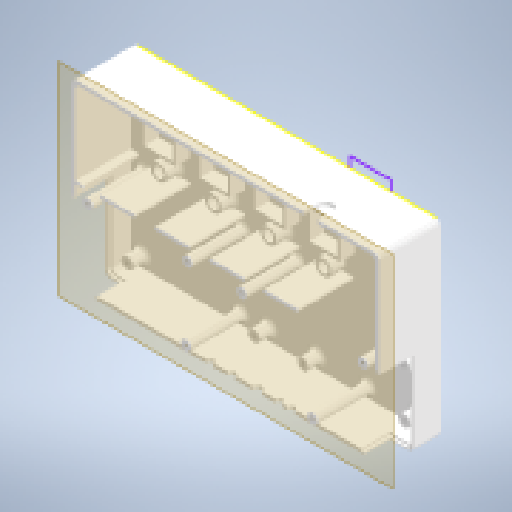
# Autodesk Inventor part: RV_ES_Bottom
Saved by Autodesk Inventor 2024.2 (Build 282272000, 272)
## iProperties
Created: 2023-07-31
Part Number: RV_ES_Bottom
Material: PC/ABS Plastic
Document SubType Name: Modeling
Designer: atrus
Density: 0.357273 g/cm^3
Appearance: Smooth - White
Mass: 71.7319 g
Surface Area: 1331.28 cm^2
Volume: 200.776 cm^3
Author: atrus
Autodesk Inventor part; units mm, degrees
ref_plane "YZ Plane" through (0, 0, 0) normal (1, 0, 0) x (0, 1, 0)
sketch "Sketch1" plane through (0, 0, 0) normal (0, 0, 1) x (1, 0, 0)
  line L0 (0, 0) -> (215.9, 0)
  line L1 (215.9, 0) -> (215.9, 132.08)
  line L2 (215.9, 132.08) -> (0, 132.08)
  line L3 (0, 132.08) -> (0, 0)
  dimension "d0" = 215.9
  dimension "d1" = 132.08
  constraints: 8 end point, 2 parallel, 1 horizontal, 1 perpendicular
  measures "d0" distance of L1.end L2.end
  measures "d1" distance of L0.end L1.end
extrude "BasePlate" add sketch "Sketch1" along normal blind 4
sketch "Sketch2" plane through (0, 0, 4) normal (0, 0, 1) x (1, 0, 0)
  circle A0 centre (10.16, 10.16) radius 1.7 construction
  circle A1 centre (99.06, 10.16) radius 1.7 construction
  circle A2 centre (133.35, 10.16) radius 1.7 construction
  circle A3 centre (204.47, 11.43) radius 1.7 construction
  circle A4 centre (156.21, 123.19) radius 1.7 construction
  circle A5 centre (123.19, 123.19) radius 1.7 construction
  circle A6 centre (80.01, 123.19) radius 1.7 construction
  circle A7 centre (46.99, 123.134) radius 1.7 construction
  circle A8 centre (10.16, 10.16) radius 4
  circle A9 centre (99.06, 10.16) radius 4
  circle A10 centre (133.35, 10.16) radius 4
  circle A11 centre (204.47, 11.43) radius 4
  circle A12 centre (156.21, 123.19) radius 4
  circle A13 centre (123.19, 123.19) radius 4
  circle A14 centre (80.01, 123.19) radius 4
  circle A15 centre (46.99, 123.134) radius 4
  circle A16 centre (8.89, 123.19) radius 1.7 construction
  circle A17 centre (8.89, 123.19) radius 4
  circle A18 centre (204.47, 44.45) radius 4
  circle A19 centre (204.47, 44.45) radius 1.7 construction
  point P0 (0, 0)
  dimension "d4" = 8
  constraints: 11 centre point, 9 equal radius, 1 coincident, 2 other
  measures "d4" diameter of A8
ref_plane "Work Plane1" through (5.1378, 6.7962, 14) normal (0, 0, 1) x (0.0000001, 1, 0)
extrude "PCB Screw Bosses" add sketch "Sketch2" along normal up to surface (10 mm away)
sketch "Sketch3" plane through (0, 0, 4) normal (0, 0, 1) x (1, 0, 0)
  line L0 (0, 0) -> (215.9, 0)
  line L1 (215.9, 0) -> (215.9, 132.08)
  line L2 (215.9, 132.08) -> (0, 132.08)
  line L3 (0, 132.08) -> (0, 0)
  line L4 (213.487, 129.667) -> (213.487, 2.413)
  line L5 (213.487, 2.413) -> (2.413, 2.413)
  line L6 (2.413, 2.413) -> (2.413, 129.667)
  line L7 (2.413, 129.667) -> (213.487, 129.667)
  point P0 (0, 132.08)
  point P1 (215.9, 0)
  dimension "d7" = 2.413
  constraints: 16 end point, 4 parallel, 2 perpendicular, 1 horizontal, 3 other
  measures "d7" distance between parallel lines of L1 L4
extrude "OuterCaseWall" add sketch "Sketch3" along normal blind 15.24
sketch "Sketch4" plane through (0, 0, 4) normal (0, 0, 1) x (1, 0, 0)
  line L0 (2.413, 129.667) -> (2.413, 2.413) projected
  line L1 (2.413, 129.667) -> (213.487, 129.667) projected
  line L2 (43.1672, 85.3312) -> (20.8152, 85.3312) construction
  line L3 (19.2531, 110.0327) -> (44.7547, 110.0327) construction
  line L4 (19.2531, 84.5311) -> (19.2531, 110.0327) construction
  line L5 (44.7547, 110.0327) -> (44.7547, 84.5311) construction
  line L6 (57.6071, 84.5311) -> (57.6071, 110.0327) construction
  line L7 (81.5212, 85.3312) -> (59.1692, 85.3312) construction
  line L8 (83.1087, 110.0327) -> (83.1087, 84.5311) construction
  line L9 (57.6071, 110.0327) -> (83.1087, 110.0327) construction
  line L10 (96.2151, 110.0327) -> (121.7167, 110.0327) construction
  line L11 (121.7167, 110.0327) -> (121.7167, 84.5311) construction
  line L12 (96.2151, 84.5311) -> (96.2151, 110.0327) construction
  line L13 (120.1292, 85.3312) -> (97.7772, 85.3312) construction
  line L14 (158.7372, 85.3312) -> (136.3852, 85.3312) construction
  line L15 (134.8231, 84.5311) -> (134.8231, 110.0327) construction
  line L16 (134.8231, 110.0327) -> (160.3247, 110.0327) construction
  line L17 (160.3247, 110.0327) -> (160.3247, 84.5311) construction
  line L18 (20.2531, 85.5311) -> (43.7547, 85.5311)
  line L19 (43.7547, 85.5311) -> (43.7547, 109.0327)
  line L20 (43.7547, 109.0327) -> (20.2531, 109.0327)
  line L21 (20.2531, 109.0327) -> (20.2531, 85.5311)
  line L22 (41.7547, 107.0327) -> (22.2531, 107.0327)
  line L23 (22.2531, 107.0327) -> (22.2531, 87.5311)
  line L24 (22.2531, 87.5311) -> (41.7547, 87.5311)
  line L25 (41.7547, 87.5311) -> (41.7547, 107.0327)
  line L26 (58.8611, 109.0327) -> (58.8611, 85.5311)
  line L27 (60.8611, 107.0327) -> (60.8611, 87.5311)
  line L28 (80.3627, 107.0327) -> (60.8611, 107.0327)
  line L29 (82.3627, 109.0327) -> (58.8611, 109.0327)
  line L30 (80.3627, 87.5311) -> (80.3627, 107.0327)
  line L31 (82.3627, 85.5311) -> (82.3627, 109.0327)
  line L32 (60.8611, 87.5311) -> (80.3627, 87.5311)
  line L33 (58.8611, 85.5311) -> (82.3627, 85.5311)
  line L34 (97.4691, 109.0327) -> (97.4691, 85.5311)
  line L35 (99.4691, 107.0327) -> (99.4691, 87.5311)
  line L36 (118.9707, 107.0327) -> (99.4691, 107.0327)
  line L37 (120.9707, 109.0327) -> (97.4691, 109.0327)
  line L38 (118.9707, 87.5311) -> (118.9707, 107.0327)
  line L39 (120.9707, 85.5311) -> (120.9707, 109.0327)
  line L40 (99.4691, 87.5311) -> (118.9707, 87.5311)
  line L41 (97.4691, 85.5311) -> (120.9707, 85.5311)
  line L42 (136.0771, 109.0327) -> (136.0771, 85.5311)
  line L43 (138.0771, 107.0327) -> (138.0771, 87.5311)
  line L44 (157.5787, 107.0327) -> (138.0771, 107.0327)
  line L45 (159.5787, 109.0327) -> (136.0771, 109.0327)
  line L46 (157.5787, 87.5311) -> (157.5787, 107.0327)
  line L47 (159.5787, 85.5311) -> (159.5787, 109.0327)
  line L48 (138.0771, 87.5311) -> (157.5787, 87.5311)
  line L49 (136.0771, 85.5311) -> (159.5787, 85.5311)
  point P0 (0, 0)
  point P1 (19.2531, 97.2819)
  dimension "d138" = 2
  dimension "d139" = 1
  dimension "d140" = 1
  dimension "d141" = 2
  dimension "d142" = 2
  dimension "d143" = 1
  dimension "d146" = 38.608
  constraints: 64 end point, 4 parallel, 4 perpendicular, 3 horizontal, 1 midpoint, 48 other
  measures "d138" distance between parallel lines of L21 L23
  measures "d139" distance between parallel lines of L5 L19
  measures "d140" distance between parallel lines of L3 L20
  measures "d141" distance between parallel lines of L19 L25
  measures "d142" distance between parallel lines of L20 L22
  measures "d143" distance from line of point (19.253, 97.282) L21
  measures "d146" distance of L20.end L26.start
extrude "ReceptBottomRibs" add sketch "Sketch4" along normal up to surface (10 mm away)
sketch "Sketch5" plane through (0, 0, 4) normal (0, 0, 1) x (1, 0, 0)
  line L0 (2.413, 129.667) -> (2.413, 2.413) projected
  line L1 (2.413, 2.413) -> (2.413, 129.667) projected
  arc A0 (157.758, 68.35) -> (157.758, 71.35) centre (157.758, 69.85) ccw construction
  line L2 (135.358, 71.35) -> (157.758, 71.35) construction
  line L3 (157.758, 68.35) -> (135.358, 68.35) construction
  arc A1 (135.358, 71.35) -> (135.358, 68.35) centre (135.358, 69.85) ccw construction
  arc A2 (120.166, 68.35) -> (120.166, 71.35) centre (120.166, 69.85) ccw construction
  line L4 (97.766, 71.35) -> (120.166, 71.35) construction
  line L5 (120.166, 68.35) -> (97.766, 68.35) construction
  arc A3 (97.766, 71.35) -> (97.766, 68.35) centre (97.766, 69.85) ccw construction
  line L6 (59.158, 71.35) -> (81.558, 71.35) construction
  line L7 (81.558, 68.35) -> (59.158, 68.35) construction
  arc A4 (59.158, 71.35) -> (59.158, 68.35) centre (59.158, 69.85) ccw construction
  arc A5 (81.558, 68.35) -> (81.558, 71.35) centre (81.558, 69.85) ccw construction
  arc A6 (20.804, 71.35) -> (20.804, 68.35) centre (20.804, 69.85) ccw construction
  line L8 (43.204, 68.35) -> (20.804, 68.35) construction
  line L9 (20.804, 71.35) -> (43.204, 71.35) construction
  arc A7 (43.204, 68.35) -> (43.204, 71.35) centre (43.204, 69.85) ccw construction
  line L10 (8.8811, 71.12) -> (8.8811, 68.58) construction
  line L11 (3.81, 71.12) -> (8.8811, 71.12) construction
  line L12 (8.8811, 68.58) -> (3.81, 68.58) construction
  line L13 (135.358, 68.75) -> (157.758, 68.75)
  arc A8 (157.758, 68.75) -> (157.758, 70.95) centre (157.758, 69.85) ccw
  line L14 (157.758, 70.95) -> (135.358, 70.95)
  arc A9 (135.358, 70.95) -> (135.358, 68.75) centre (135.358, 69.85) ccw
  line L15 (97.766, 68.75) -> (120.166, 68.75)
  arc A10 (120.166, 68.75) -> (120.166, 70.95) centre (120.166, 69.85) ccw
  line L16 (120.166, 70.95) -> (97.766, 70.95)
  arc A11 (97.766, 70.95) -> (97.766, 68.75) centre (97.766, 69.85) ccw
  line L17 (59.158, 68.75) -> (81.558, 68.75)
  arc A12 (81.558, 68.75) -> (81.558, 70.95) centre (81.558, 69.85) ccw
  line L18 (81.558, 70.95) -> (59.158, 70.95)
  arc A13 (59.158, 70.95) -> (59.158, 68.75) centre (59.158, 69.85) ccw
  arc A14 (20.804, 70.95) -> (20.804, 68.75) centre (20.804, 69.85) ccw
  line L19 (20.804, 70.95) -> (43.204, 70.95)
  arc A15 (43.204, 68.75) -> (43.204, 70.95) centre (43.204, 69.85) ccw
  line L20 (43.204, 68.75) -> (20.804, 68.75)
  line L21 (2.413, 70.72) -> (8.4811, 70.72)
  line L22 (8.4811, 70.72) -> (8.4811, 68.98)
  line L23 (8.4811, 68.98) -> (2.413, 68.98)
  line L24 (2.413, 68.98) -> (2.413, 70.72)
  point P0 (0, 0)
  point P1 (2.413, 87.122)
  point P2 (5.447, 68.98)
  point P3 (5.447, 70.72)
  point P4 (8.8811, 69.85)
  point P5 (8.4811, 69.85)
  point P6 (2.413, 69.85)
  dimension "d134" = 0.4
  dimension "d135" = 0.4
  dimension "d136" = 0.4
  dimension "d137" = 0.4
  constraints: 46 end point, 32 point on circle, 16 centre point, 11 horizontal, 5 midpoint, 3 collinear, 2 parallel, 1 perpendicular, 1 point on line, 1 vertical, 48 other
  measures "d134" distance between parallel lines of L9 L19
  measures "d135" distance from line of L12 point (5.447, 68.98)
  measures "d136" distance from line of L11 point (5.447, 70.72)
  measures "d137" distance of point (8.881, 69.85) point (8.481, 69.85)
ref_plane "Top Of Case" through (17.5673, 114.3074, 42.9916) normal (0, 0, 1) x (1, 0, 0)
ref_plane "Offset Top Of Case" through (17.5673, 114.3074, 42.7916) normal (0, 0, 1) x (1, 0, 0)
extrude "Barriers" add sketch "Sketch5" along normal up to surface (38.9916 mm away)
sketch "Sketch6" plane through (0, 0, 4) normal (0, 0, 1) x (1, 0, 0)
  circle A0 centre (29.21, 123.19) radius 3.75 projected
  circle A1 centre (90.17, 123.19) radius 3.75 projected
  circle A2 centre (113.03, 123.19) radius 3.75 projected
  circle A3 centre (181.61, 123.19) radius 3.75 projected
  circle A4 centre (29.21, 123.19) radius 5.75
  circle A5 centre (90.17, 123.19) radius 5.75
  circle A6 centre (113.03, 123.19) radius 5.75
  circle A7 centre (181.61, 123.19) radius 5.75
  circle A8 centre (194.31, 73.66) radius 5.75
  circle A9 centre (108.966, 76.2) radius 5.75
  circle A10 centre (70.358, 76.2) radius 5.75
  circle A11 centre (32.004, 76.2) radius 5.75
  circle A12 centre (194.31, 73.66) radius 3.75 projected
  circle A13 centre (108.966, 76.2) radius 3.75 projected
  circle A14 centre (32.004, 76.2) radius 3.75 projected
  circle A15 centre (70.358, 76.2) radius 3.75 projected
  circle A16 centre (147.574, 76.2) radius 3.75 projected
  circle A17 centre (147.574, 76.2) radius 5.75
  dimension "d52" = 2
  constraints: 9 centre point, 8 equal radius, 5 coincident
  measures "d52" radial gap between concentric circles of A0 A4
extrude "HVSideBosses" add sketch "Sketch6" along normal up to surface (10 mm away)
sketch "Sketch7" plane through (0, 0, 0) normal (0, 0, -1) x (-1, 0, 0)
  circle A0 centre (-29.21, 123.19) radius 3.75 projected
  circle A1 centre (-90.17, 123.19) radius 3.75 projected
  circle A2 centre (-113.03, 123.19) radius 3.75 projected
  circle A3 centre (-181.61, 123.19) radius 3.75 projected
  circle A4 centre (-32.004, 76.2) radius 3.75 projected
  circle A5 centre (-70.358, 76.2) radius 3.75 projected
  circle A6 centre (-108.966, 76.2) radius 3.75 projected
  circle A7 centre (-147.574, 76.2) radius 3.75 projected
  circle A8 centre (-194.31, 73.66) radius 3.75 projected
  point P0 (0, 0)
  constraints: 5 coincident
hole "HotSideHoles" at (29.21, 123.19, 0) at (90.17, 123.19, 0) at (113.03, 123.19, 0) at (181.61, 123.19, 0) at (194.31, 73.66, 0) at (32.004, 76.2, 0) at (70.358, 76.2, 0) at (108.966, 76.2, 0) at (147.574, 76.2, 0) direction (0, 0, 1) diameter 3.2766 end through all counterbore diameter 7.62 counterbore depth 3 clearance for "Flat Head Machine Screw (82)" size "#4" standard "Ansi Unified Screw Threads"
chamfer "HotSideHoleChamfer" distance 2.032 angle 45 9 edges at (90.17, 119.38, 3) (113.03, 119.38, 3) (181.61, 119.38, 3) (29.21, 119.38, 3) (194.31, 69.85, 3) (32.004, 72.39, 3) (70.358, 72.39, 3) (108.966, 72.39, 3) (147.574, 72.39, 3)
sketch "Sketch8" plane through (0, 0, 4) normal (0, 0, 1) x (1, 0, 0)
  circle A0 centre (169.052, 9.398) radius 3.45
  circle A1 centre (80.01, 9.398) radius 3.45
  circle A2 centre (81.28, 60.96) radius 3.45
  circle A3 centre (119.38, 60.96) radius 3.45
  circle A4 centre (204.47, 60.96) radius 3.45
  circle A5 centre (11.43, 60.96) radius 3.45
  circle A6 centre (169.052, 9.398) radius 3.75 projected
  circle A7 centre (80.01, 9.398) radius 3.75 projected
  circle A8 centre (119.38, 60.96) radius 3.75 projected
  circle A9 centre (81.28, 60.96) radius 3.75 projected
  circle A10 centre (204.47, 60.96) radius 3.75 projected
  circle A11 centre (11.43, 60.96) radius 3.75 projected
  point P0 (0, 0)
  constraints: 6 centre point, 6 coincident, 5 equal radius
extrude "LogicSideBosses" add sketch "Sketch8" along normal up to surface (38.9916 mm away) contours A0 | A1 | A2 | A3 | A4 | A5
sketch "Sketch9" plane through (81.28, 60.96, 42.9916) normal (0, 0, 1) x (1, 0, 0)
  circle A0 centre (-69.85, 0) radius 3.45 construction
  circle A1 centre (0, 0) radius 3.45 construction
  circle A2 centre (38.1, 0) radius 3.45 construction
  circle A3 centre (123.19, 0) radius 3.45 construction
  circle A4 centre (87.772, -51.562) radius 3.45 construction
  circle A5 centre (17.78, -50.8) radius 4
  circle A6 centre (-1.27, -51.562) radius 3.45 construction
  point P0 (-81.28, -60.96)
  constraints: 1 centre point
hole "LogicSideHoles" at (11.43, 60.96, 42.9916) at (81.28, 60.96, 42.9916) at (119.38, 60.96, 42.9916) at (204.47, 60.96, 42.9916) at (169.052, 9.398, 42.9916) at (80.01, 9.398, 42.9916) direction (0, 0, -1) diameter 2.1565 depth 17.78 tip angle 118 thread size "4-40 UNC" class "2B" standard "ANSI Unified Screw Threads"
fillet "Fillet1" radius 3.175 21 edges at (7.98, 60.96, 4) (77.83, 60.96, 4) (115.93, 60.96, 4) (76.56, 9.398, 4) (165.602, 9.398, 4) (201.02, 60.96, 4) (108.966, 81.95, 4) (70.358, 81.95, 4) (32.004, 81.95, 4) (42.99, 123.134, 4) (76.01, 123.19, 4) (119.19, 123.19, 4) (4.89, 123.19, 4) (175.86, 123.19, 4) (152.21, 123.19, 4) (23.46, 123.19, 4) (6.16, 10.16, 4) (95.06, 10.16, 4) (129.35, 10.16, 4) (200.47, 11.43, 4) (200.47, 44.45, 4)
sketch "Sketch10" plane through (46.99, 123.134, 14) normal (0, 0, 1) x (1, 0, 0)
  circle A0 centre (-38.1, 0.056) radius 4 projected
  circle A1 centre (0, 0) radius 4 projected
  circle A2 centre (33.02, 0.056) radius 4 projected
  circle A3 centre (76.2, 0.056) radius 4 projected
  circle A4 centre (109.22, 0.056) radius 4 projected
  circle A5 centre (157.48, -111.704) radius 4 projected
  circle A6 centre (86.36, -112.974) radius 4 projected
  circle A7 centre (52.07, -112.974) radius 4 projected
  circle A8 centre (-36.83, -112.974) radius 4 projected
  line L0 (-44.577, -120.721) -> (166.497, -120.721) projected
  line L1 (166.497, -120.721) -> (166.497, 6.533) projected
  line L2 (166.497, 6.533) -> (140.7604, 6.533) projected
  circle A9 centre (147.32, -49.474) radius 5.75 projected
  circle A10 centre (157.48, -78.684) radius 1.7 projected
  line L3 (-44.577, 6.533) -> (-44.577, 3.1429) projected
  arc A11 (39.0064, -3.8992) -> (39.0064, 4.0112) centre (43.18, 0.056) ccw projected
  arc A12 (70.2136, 4.0112) -> (70.2136, -3.8992) centre (66.04, 0.056) ccw projected
  line L4 (-44.577, -54.154) -> (-44.577, -120.721) projected
  arc A13 (29.9331, 6.533) -> (39.0064, -3.8992) centre (33.02, 0.056) ccw projected
  line L5 (29.9331, 6.533) -> (2.9666, 6.533) projected
  arc A14 (-2.9666, 6.533) -> (2.9666, 6.533) centre (0, 0) ccw projected
  arc A15 (73.1131, 6.533) -> (70.2136, 4.0112) centre (76.2, 0.056) ccw projected
  line L6 (73.1131, 6.533) -> (36.1069, 6.533) projected
  arc A16 (39.0064, 4.0112) -> (36.1069, 6.533) centre (33.02, 0.056) ccw projected
  arc A17 (-41.1869, 6.533) -> (-44.577, 3.1429) centre (-38.1, 0.056) ccw projected
  line L7 (-41.1869, 6.533) -> (-44.577, 6.533) projected
  arc A18 (-44.577, -3.0309) -> (-35.0131, 6.533) centre (-38.1, 0.056) ccw projected
  arc A19 (-23.9204, 6.533) -> (-11.6396, 6.533) centre (-17.78, 0.056) ccw projected
  line L8 (-2.9666, 6.533) -> (-11.6396, 6.533) projected
  line L9 (-23.9204, 6.533) -> (-35.0131, 6.533) projected
  circle A20 centre (-36.83, -112.974) radius 7.175 projected
  arc A21 (128.4796, 6.533) -> (140.7604, 6.533) centre (134.62, 0.056) ccw projected
  line L10 (128.4796, 6.533) -> (112.3069, 6.533) projected
  arc A22 (106.1331, 6.533) -> (112.3069, 6.533) centre (109.22, 0.056) ccw projected
  arc A23 (30.5856, -52.184) -> (16.1504, -52.184) centre (23.368, -46.934) ccw projected
  circle A24 centre (157.48, -62.174) radius 6.625 projected
  arc A25 (69.1936, -52.184) -> (54.7584, -52.184) centre (61.976, -46.934) ccw projected
  arc A26 (-7.7684, -52.184) -> (-22.2036, -52.184) centre (-14.986, -46.934) ccw projected
  line L11 (-44.577, -3.0309) -> (-44.577, -52.414) projected
  line L12 (106.1331, 6.533) -> (79.2869, 6.533) projected
  arc A27 (70.2136, -3.8992) -> (79.2869, 6.533) centre (76.2, 0.056) ccw projected
  line L13 (-44.577, -52.414) -> (-38.5089, -52.414) projected
  line L14 (-38.5089, -52.414) -> (-38.5089, -54.154) projected
  line L15 (-38.5089, -54.154) -> (-44.577, -54.154) projected
  line L16 (69.1936, -52.184) -> (73.176, -52.184) projected
  arc A28 (73.176, -54.384) -> (73.176, -52.184) centre (73.176, -53.284) ccw projected
  line L17 (73.176, -54.384) -> (50.776, -54.384) projected
  arc A29 (50.776, -52.184) -> (50.776, -54.384) centre (50.776, -53.284) ccw projected
  line L18 (50.776, -52.184) -> (54.7584, -52.184) projected
  line L19 (30.5856, -52.184) -> (34.568, -52.184) projected
  arc A30 (34.568, -54.384) -> (34.568, -52.184) centre (34.568, -53.284) ccw projected
  line L20 (34.568, -54.384) -> (12.168, -54.384) projected
  arc A31 (12.168, -52.184) -> (12.168, -54.384) centre (12.168, -53.284) ccw projected
  line L21 (12.168, -52.184) -> (16.1504, -52.184) projected
  line L22 (-7.7684, -52.184) -> (-3.786, -52.184) projected
  arc A32 (-3.786, -54.384) -> (-3.786, -52.184) centre (-3.786, -53.284) ccw projected
  line L23 (-3.786, -54.384) -> (-26.186, -54.384) projected
  arc A33 (-26.186, -52.184) -> (-26.186, -54.384) centre (-26.186, -53.284) ccw projected
  line L24 (-26.186, -52.184) -> (-22.2036, -52.184) projected
  point P0 (-46.99, -123.134)
hole "PCBMountHoles" at (46.99, 123.134, 14) at (8.89, 123.19, 14) at (80.01, 123.19, 14) at (123.19, 123.19, 14) at (156.21, 123.19, 14) at (10.16, 10.16, 14) at (99.06, 10.16, 14) at (133.35, 10.16, 14) at (204.47, 11.43, 14) at (204.47, 44.45, 14) direction (0, 0, -1) diameter 2.1565 end through all thread size "4-40 UNC" class "2B" standard "ANSI Unified Screw Threads"
sketch "Sketch11" plane through (0, 0, 19.24) normal (0, 0, 1) x (1, 0, 0)
  line L0 (2.413, 59.24) -> (2.413, 129.667) projected
  line L1 (2.413, 59.24) -> (2.413, 129.667)
  line L2 (2.413, 129.667) -> (213.487, 129.667) projected
  line L3 (2.413, 129.667) -> (213.487, 129.667)
  line L4 (213.487, 129.667) -> (213.487, 59.24)
  line L5 (213.487, 129.667) -> (213.487, 2.413) projected
  line L6 (215.9, 0) -> (215.9, 132.08) projected
  line L7 (215.9, 59.24) -> (215.9, 132.08)
  line L8 (215.9, 132.08) -> (0, 132.08)
  line L9 (0, 132.08) -> (0, 59.24)
  line L10 (0, 132.08) -> (0, 0) projected
  line L11 (2.413, 59.24) -> (0, 59.24)
  line L12 (213.487, 59.24) -> (215.9, 59.24)
  point P0 (2.413, 66.4695)
  point P1 (1.2065, 59.24)
  dimension "d120" = 72.84
  constraints: 16 end point, 3 point on line, 2 horizontal, 2 horizontal alignment, 2 vertical, 1 collinear, 1 midpoint, 1 perpendicular
  measures "d120" distance from line of L8 point (1.206, 59.24)
extrude "HV Upper Wall" add sketch "Sketch11" along normal up to surface (23.7516 mm away)
fillet "HV Corner Fillets" radius 3.175 4 edges at (0, 132.08, 21.4958) (213.487, 129.667, 23.4958) (215.9, 132.08, 21.4958) (2.413, 129.667, 23.4958)
sketch "Sketch13" plane through (194.31, 73.66, 14) normal (0, 0, 1) x (1, 0, 0)
  line L0 (-65.5099, -5.6483) -> (-65.5099, -7.1905) construction
  line L1 (19.177, -71.247) -> (19.177, 52.832) construction
  line L2 (-4.3589, -19.325) -> (-4.3589, -3.75)
  line L3 (-4.3589, -3.75) -> (4.3589, -3.75)
  line L4 (4.3589, -3.75) -> (4.3589, -19.325)
  line L5 (4.3589, -19.325) -> (-4.3589, -19.325)
  arc A0 (-5.75, 0) -> (-5.75, 0) centre (0, 0) ccw projected
  circle A1 centre (0, 0) radius 3.75 projected
  arc A2 (16.785, -12.7) -> (16.785, -12.7) centre (10.16, -12.7) ccw construction
  point P0 (-194.31, -73.66)
  point P1 (0, -3.75)
  constraints: 8 end point, 2 point on circle, 2 vertical, 1 midpoint, 1 parallel, 1 perpendicular, 1 tangent, 1 vertical alignment, 1 other
extrude "BossCutPowerSupply" cut sketch "Sketch13" against normal up to surface (10 mm away) contours L2 A0 L4 L5 | L3 A0 picked at (2.5581, -4.066)
fillet "LgicCornerFillets" radius 3.175 4 edges at (0, 0, 9.62) (215.9, 0, 9.62) (2.413, 2.413, 11.62) (213.487, 2.413, 11.62)
sketch "Sketch14" plane through (0, 0, 19.24) normal (0, 0, 1) x (1, 0, 0)
  circle A0 centre (80.01, 9.398) radius 1.0782 construction
  circle A1 centre (80.01, 9.398) radius 3.45 construction
  line L0 (151.92, 16.9397) -> (151.92, 21.3401) construction
  line L1 (84.975, 21.3101) -> (84.975, 16.9097) construction
  line L2 (5.588, 2.413) -> (210.312, 2.413) projected
  line L3 (3.175, 0) -> (212.725, 0) projected
  line L4 (10.668, 2.413) -> (199.39, 2.413)
  line L5 (199.39, 2.413) -> (199.39, 0)
  line L6 (199.39, 0) -> (10.668, 0)
  line L7 (10.668, 0) -> (10.668, 2.413)
  circle A2 centre (204.47, 11.43) radius 1.0782 construction
  point P0 (0, 0)
  point P1 (199.39, 1.2065)
  point P2 (151.92, 19.1399)
  point P3 (10.668, 1.2065)
  point P4 (84.975, 19.1099)
  point P5 (10.668, 0)
  point P6 (199.39, 2.413)
  dimension "d95" = 5.08
  dimension "d96" = 5.08
  constraints: 8 end point, 4 midpoint, 2 parallel, 2 point on line, 1 horizontal, 1 perpendicular
  measures "d95" horizontal distance of point (199.39, 1.206) A2.centre
  measures "d96" horizontal distance of L2.start point (10.668, 1.206)
extrude "Extrusion11" add sketch "Sketch14" along normal blind 17.78
sketch "Sketch15" plane through (3.175, 0, 0) normal (0, -1, 0) x (1, 0, 0)
  line L0 (7.493, 37.02) -> (196.215, 37.02) projected
  circle A0 centre (88.11, 37.02) radius 2.54
  circle A1 centre (103.2, 37.02) radius 2.54
  circle A2 centre (120.915, 37.02) radius 3.175
  circle A3 centre (136.155, 37.02) radius 2.54
  circle A4 centre (144.945, 37.02) radius 2.54
  line L1 (88.26, 22.2733) -> (89.674, 22.2733) construction
  ellipse E0 centre (88.86, 23.1218) end of major axis (90.31, 23.1218) minor radius 1.0253 (89.674, 22.2733) -> (89.76, 22.3179) ccw construction
  line L2 (89.76, 22.3179) -> (89.76, 23.9257) construction
  ellipse E1 centre (88.86, 23.1218) end of major axis (90.31, 23.1218) minor radius 1.0253 (89.76, 23.9257) -> (89.674, 23.9704) ccw construction
  line L3 (89.674, 23.9704) -> (88.86, 23.9704) construction
  line L4 (88.86, 23.9704) -> (88.26, 23.9704) construction
  line L5 (88.26, 23.9704) -> (88.26, 22.2733) construction
  line L6 (103.5, 22.2733) -> (104.914, 22.2733) construction
  ellipse E2 centre (104.1, 23.1218) end of major axis (105.55, 23.1218) minor radius 1.0253 (104.914, 22.2733) -> (105, 22.3179) ccw construction
  line L7 (105, 22.3179) -> (105, 23.9257) construction
  ellipse E3 centre (104.1, 23.1218) end of major axis (105.55, 23.1218) minor radius 1.0253 (105, 23.9257) -> (104.914, 23.9704) ccw construction
  line L8 (104.914, 23.9704) -> (104.1, 23.9704) construction
  line L9 (104.1, 23.9704) -> (103.5, 23.9704) construction
  line L10 (103.5, 23.9704) -> (103.5, 22.2733) construction
  line L11 (140.115, 28.8269) -> (137.325, 28.8269) construction
  point P0 (-3.175, 0)
  point P1 (144.945, 28.8269)
  point P2 (88.11, 26.7147)
  point P3 (103.2, 27.1269)
  point P4 (120.915, 27.1269)
  point P5 (136.155, 26.6735)
  point P6 (147.485, 37.02)
  point P7 (142.405, 37.02)
  point P8 (124.09, 37.02)
  point P9 (117.74, 37.02)
  point P10 (105.74, 37.02)
  point P11 (100.66, 37.02)
  point P12 (90.65, 37.02)
  point P13 (85.57, 37.02)
  dimension "d90" = 5.08
  dimension "d91" = 6.35
  dimension "d92" = 5.08
  constraints: 5 centre point, 5 point on line, 5 vertical alignment, 2 equal radius, 10 other
  measures "d90" diameter of A0
  measures "d91" diameter of A2
  measures "d92" diameter of A3
extrude "Extrusion12" cut sketch "Sketch15" against normal blind 19.05 contours L0 A0 | L0 A1 | L0 A2 | A3 L0 | L0 A3 | L0 A4 picked at (88.2121, 36.1795) picked at (103.3021, 36.1795) picked at (120.0921, 36.0649) picked at (144.3481, 35.3683)
sketch "Sketch16" plane through (0, 0, 19.24) normal (0, 0, 1) x (1, 0, 0)
  line L0 (10.668, 2.413) -> (5.588, 2.413) projected
  arc A0 (2.413, 5.588) -> (5.588, 2.413) centre (5.588, 5.588) ccw projected
  line L1 (2.413, 5.588) -> (2.413, 59.24) projected
  line L2 (1.113, 59.24) -> (1.113, 5.588)
  arc A1 (1.113, 5.588) -> (5.588, 1.113) centre (5.588, 5.588) ccw
  line L3 (5.588, 1.113) -> (10.668, 1.113)
  line L4 (2.413, 59.24) -> (0, 59.24) projected
  line L5 (1.113, 59.24) -> (2.413, 59.24)
  line L6 (10.668, 0) -> (10.668, 2.413) projected
  line L7 (10.668, 2.413) -> (10.668, 1.113)
  line L8 (213.487, 59.24) -> (213.487, 5.588) projected
  arc A2 (210.312, 2.413) -> (213.487, 5.588) centre (210.312, 5.588) ccw projected
  line L9 (210.312, 2.413) -> (199.39, 2.413) projected
  line L10 (214.787, 59.24) -> (214.787, 5.588)
  arc A3 (210.312, 1.113) -> (214.787, 5.588) centre (210.312, 5.588) ccw
  line L11 (210.312, 1.113) -> (199.39, 1.113)
  line L12 (215.9, 59.24) -> (213.487, 59.24) projected
  line L13 (214.787, 59.24) -> (213.487, 59.24)
  line L14 (199.39, 1.113) -> (199.39, 2.413)
  line L15 (5.588, 2.413) -> (210.312, 2.413) projected
  point P0 (0, 0)
  dimension "d97" = 1.3
  dimension "d100" = 1.3
  constraints: 16 end point, 4 point on circle, 2 centre point, 2 perpendicular, 1 collinear, 1 horizontal, 4 other
  measures "d97" distance between parallel lines of L1 L2
  measures "d100" distance between parallel lines of L8 L10
extrude "OuterWallLip" cut sketch "Sketch16" against normal blind 2
sketch "Sketch17" plane through (0, 59.24, 42.9916) normal (0, -1, 0) x (1, 0, 0)
  line L0 (214.787, -23.7516) -> (214.787, -25.7516) projected
  line L1 (214.787, -23.7516) -> (214.7559, 0)
  line L2 (215.9, 0) -> (213.487, 0) projected
  line L3 (214.7559, 0) -> (213.487, 0)
  line L4 (213.487, 0) -> (213.487, -25.7516)
  line L5 (213.487, -25.7516) -> (214.787, -25.7516)
  line L6 (214.787, -23.7516) -> (214.787, -25.7516)
  line L7 (1.113, -25.7516) -> (2.413, -25.7516) projected
  line L8 (1.113, -25.7516) -> (2.413, -25.7516)
  line L9 (2.413, 0) -> (2.413, -25.7516) projected
  line L10 (2.413, -25.7516) -> (2.413, 0)
  line L11 (1.113, -23.7516) -> (1.113, -25.7516) projected
  line L12 (1.113, -25.7516) -> (1.113, -23.7516)
  line L13 (1.113, -23.7516) -> (1.113, 0)
  line L14 (2.413, 0) -> (0, 0) projected
  line L15 (2.413, 0) -> (1.113, 0)
  point P0 (0, -42.9916)
  constraints: 20 end point, 4 perpendicular, 3 point on line, 1 collinear, 1 horizontal, 1 vertical
extrude "Extrusion14" cut sketch "Sketch17" against normal blind 2
sketch "Sketch18" plane through (199.39, 0, 37.02) normal (1, 0, 0) x (0, 0, -1)
  line L0 (17.78, 1.113) -> (19.78, 1.113) projected
  line L1 (19.78, 1.113) -> (19.78, 2.413) projected
  line L2 (17.78, 1.113) -> (17.78, 0) projected
  line L3 (0, 2.413) -> (19.78, 2.413) projected
  line L4 (19.78, 2.413) -> (0, 2.413)
  line L5 (17.78, 1.113) -> (0, 1.113)
  line L6 (0, 0) -> (0, 2.413) projected
  line L7 (0, 2.413) -> (0, 1.113)
  point P0 (37.02, 0)
  constraints: 6 end point, 1 horizontal, 1 perpendicular, 1 point on line
extrude "Extrusion15" cut sketch "Sketch18" against normal blind 2
sketch "Sketch19" plane through (10.668, 0, 37.02) normal (-1, 0, 0) x (0, 0, 1)
  line L0 (-17.78, 1.113) -> (-19.78, 1.113) projected
  line L1 (-19.78, 2.413) -> (-19.78, 1.113) projected
  line L2 (-19.78, 2.413) -> (0, 2.413) projected
  line L3 (-17.78, 1.113) -> (0, 1.113)
  line L4 (0, 2.413) -> (0, 0) projected
  line L5 (0, 2.413) -> (0, 1.113)
  point P0 (-37.02, 0)
  constraints: 4 end point, 1 horizontal, 1 perpendicular, 1 point on line
extrude "Extrusion16" cut sketch "Sketch19" against normal blind 2
sketch "Sketch20" plane through (0, 0, 0) normal (0, 0, -1) x (-1, 0, 0)
  line L0 (-212.725, 132.08) -> (-3.175, 132.08) projected
  line L1 (-185.42, 132.08) -> (-185.42, 137.16)
  line L2 (-185.42, 137.16) -> (-150.0124, 137.16)
  line L3 (-150.0124, 137.16) -> (-150.0124, 132.08)
  line L4 (-215.9, 3.175) -> (-215.9, 128.905) projected
  line L5 (-213.487, 61.24) -> (-213.487, 126.492) projected
  point P0 (0, 0)
  point P1 (-185.42, 134.62)
  dimension "d151" = 5.08
  dimension "d153" = 35.4076
  dimension "d159" = 30.48
  constraints: 6 end point, 2 perpendicular, 2 point on line, 1 midpoint, 1 vertical
  measures "d151" distance of L1.start L1.end
  measures "d153" distance of L1.end L2.end
  measures "d159" distance from line of point (-185.42, 134.62) L4
ref_plane "Work Plane4" through (0, 59.3195, 43.0916) normal (0, 0, -1) x (0, 1, 0)
extrude "Extrusion17" add sketch "Sketch20" against normal up to surface (42.9916 mm away)
sketch "Sketch12" plane through (-1.7526, 137.16, 0) normal (0, 1, 0) x (1, 0, 0)
  line L0 (212.0646, -42.9916) -> (7.3406, -42.9916) projected
  line L1 (174.4726, -42.9916) -> (174.4726, -32.7516)
  line L2 (169.4726, -27.7516) -> (169.4726, -27.7516)
  line L3 (164.4726, -32.7516) -> (164.4726, -42.9916)
  line L4 (215.9, 0) -> (215.9, -42.9916) projected
  arc A0 (169.4726, -27.7516) -> (164.4726, -32.7516) centre (169.4726, -32.7516) ccw
  arc A1 (174.4726, -32.7516) -> (169.4726, -27.7516) centre (169.4726, -32.7516) ccw
  line L5 (217.6526, -42.9916) -> (217.6526, 0) projected
  point P0 (1.7526, 0)
  point P1 (213.487, -42.9916)
  point P2 (2.413, -42.9916)
  point P3 (174.4726, -27.7516)
  point P4 (164.4726, -27.7516)
  point P5 (174.4726, -37.8716)
  dimension "d74" = 10
  dimension "d76" = 15.24
  dimension "d77" = 5
  dimension "d158" = 43.18
  constraints: 6 end point, 6 point on line, 4 point on circle, 4 tangent, 2 centre point, 2 perpendicular, 1 concentric, 1 midpoint, 1 vertical
  measures "d74" distance of point (174.473, -27.752) point (164.473, -27.752)
  measures "d76" distance of point (164.473, -27.752) L3.end
  measures "d77" radius of A0
  measures "d158" distance between parallel lines of L1 L5
extrude "Cord cut" cut sketch "Sketch12" against normal blind 25.4
fillet "Fillet4" radius 3.175 4 edges at (185.42, 132.08, 21.4958) (150.0124, 132.08, 21.4958) (150.0124, 137.16, 21.4958) (185.42, 137.16, 21.4958)
body "Solid1"
